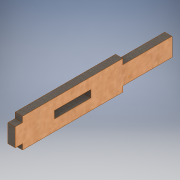
# Autodesk Inventor part: PistonPart4
Saved by Autodesk Inventor 2019 (Build 230136000, 136)
## iProperties
Created: 2021-01-03
Part Number: PistonPart4
Material: Дерево (вишня)
Document SubType Name: Modeling
Designer: Professional
Density: 0.63 g/cm^3
Appearance: Вишневое дерево — натуральный — со слабым глянцем
Author: Professional
Autodesk Inventor part; units mm, degrees
ref_plane "YZ Plane" through (0, 0, 0) normal (1, 0, 0) x (0, 1, 0)
ref_plane "XZ Plane" through (0, 0, 0) normal (0, 1, 0) x (-1, 0, 0)
ref_plane "XY Plane" through (0, 0, 0) normal (0, 0, 1) x (1, 0, 0)
sketch "Эскиз1" plane through (0, 0, 0) normal (1, 0, 0) x (0, 1, 0)
  line L0 (-8, 55) -> (8, 55) construction
  line L1 (8, 55) -> (8, 0)
  line L2 (8, 0) -> (-8, 0) construction
  line L3 (-8, 0) -> (-8, 55)
  line L4 (8, 0) -> (5, 0)
  line L5 (5, 0) -> (5, -27)
  line L6 (5, -27) -> (-5, -27)
  line L7 (-5, -27) -> (-5, 0)
  line L8 (-8, 0) -> (-5, 0)
  line L9 (0, 59) -> (0, -27) construction
  line L10 (8, 55) -> (5, 55)
  line L11 (5, 55) -> (5, 59)
  line L12 (5, 59) -> (0, 59)
  line L13 (-8, 55) -> (-5, 55)
  line L14 (-5, 55) -> (-5, 59)
  line L15 (-5, 59) -> (0, 59)
  line L16 (-2, 37.5) -> (2, 37.5)
  line L17 (2, 37.5) -> (2, 17.5)
  line L18 (2, 17.5) -> (-2, 17.5)
  line L19 (-2, 17.5) -> (-2, 37.5)
  point P0 (0, 0)
  point P1 (2, 27.5)
  point P2 (8, 27.5)
  point P3 (0, 37.5)
  dimension "d0" = 10
  dimension "d1" = 16
  dimension "d2" = 27
  dimension "d3" = 55
  dimension "d4" = 4
  dimension "d7" = 20
  dimension "d8" = 4
  constraints: 40 end point, 5 midpoint, 5 perpendicular, 5 point on line, 4 parallel, 2 horizontal, 2 symmetric about line, 2 vertical, 1 collinear, 1 horizontal alignment, 1 vertical alignment, 1 other
  measures "d0" distance between parallel lines of L5 L7
  measures "d1" distance between parallel lines of L1 L3
  measures "d2" distance between parallel lines of L6 L2
  measures "d3" distance between parallel lines of L0 L2
  measures "d4" distance of L10.end L11.end
  measures "d7" distance between parallel lines of L18 L16
  measures "d8" distance between parallel lines of L19 L17
extrude "Выдавливание2" add sketch "Эскиз1" along normal blind 4
